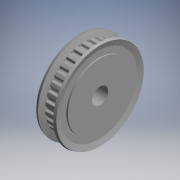
# Autodesk Inventor part: ATP30XL025-A-H10_b
Saved by Autodesk Inventor 2017.3 (Build 213256000, 256)
## iProperties
Part Number: ATP30XL025-A-H10_b
Material: Generic
Catalog Web Link: www.cadenas.de
Description: ATP__XL025, ATP__XL031, ATP__ XL037, ATP__XL050, BTP__XL025, BTP__XL031, BTP__XL037, BTP__XL050, KTP__XL025, KTP__XL031, KTP__ XL037, KTP__XL050, NTP__XL025, NTP__XL031, NTP__ XL037, NTP__XL050, MTP__XL025, MTP__ XL037, MTP__XL050, MTPB__XL025, MTPB__ XL037, MTPB__XL050, MTPP__XL025, MTPP__ XL037, MTPP__XL050, STP__XL025, STP__ XL037, STP__XL050_body-Timing Pulleys XL Type
Vendor: MISUMI
Document SubType Name: Modeling
Designer: partserver
Manufacturer: MISUMI
Mass: 21.798 g
Surface Area: 84.2967 cm^2
Volume: 21.798 cm^3
Density: 1 g/cm^3
Appearance: PSOLRGB-192-192-192
Category: PARTsolutions
Company: MISUMI
Title: ATP30XL025-A-H10
Author: Cadenas PARTsolutions
Comments: Timing Pulleys XL Type
PSOL_IDENT_0: {$CADENAS_DATA\23d-libs\misumi\metric\51_timing_pulleys\mtp_xl\mtp_xl.prj},758 {VTYP=3D},{NB=ATP30XL
PSOL_IDENT_1: 025-A-H10_b},{LINA=ATP30XL025-A-H10},{NN=ATP__XL025, ATP__XL031, ATP__ XL037, ATP__XL050, BTP__XL025
PSOL_IDENT_2: , BTP__XL031, BTP__XL037, BTP__XL050, KTP__XL025, KTP__XL031, KTP__ XL037, KTP__XL050, NTP__XL025, N
PSOL_IDENT_3: TP__XL031, NTP__ XL037, NTP__XL050, MTP__XL025, MTP__ XL037, MTP__XL050, MTPB__XL025, MTPB__ XL037,
PSOL_IDENT_4: MTPB__XL050, MTPP__XL025, MTPP__ XL037, MTPP__XL050, STP__XL025, STP__ XL037, STP__XL050_body},{DATE=
PSOL_IDENT_5: 18.04.2019 05:28:45},{GEOMDATE=08.04.2019 09:29:40},{VERSION=},{LINEID=160},{WBVAR=MATP,ST,TNW,PS,SB
PSOL_IDENT_6: S,DD,Z,J,Q,R,S,T,ALT1,ALT2,M,QSC,QFC,QTC,ALT3,K,KSC,KFC,KTC,ALT4,ZM,ZSC,ZFC,ZTC,ALT5,ALT6,ALT7,FC,AL
PSOL_IDENT_7: T8,SRG,ALT9,BTC,TL,ALT10,TPC,ALT11,BC,ALT12,SLH},{WBNUMERIC=DD,Z,J,Q,R,S,T,QSC,QFC,QTC,K,KSC,KFC,KTC
PSOL_IDENT_8: ,ZSC,ZFC,ZTC,FC,SRG,BTC,TL,BC,SLH}  {NB=ATP30XL025-A-H10_b},{LINA=ATP30XL025-A-H10},{KT=DUMMY},{PN=A
PSOL_IDENT_9: TP30XL025-A-H10},{TYPE=ATP},{MATP=A2017},{MATPALG= 'A2017','Aluminum Alloy 2000 series','S45C','1045
PSOL_IDENT_10: Carbon Steel Equivalent','SUS304','SUS304' },{ST=CA},{STALG= 'CA','Clear Anodize','BA','Black Anodi
PSOL_IDENT_11: ze','HAT','Hard Clear Anodize','ENP','Electroless Nickel Plating' },{NT=30},{TNW=XL025},{TNWALG= 'XL
PSOL_IDENT_12: 025','XL031','XL037','XL050' },{BW=6.4mm (1/4inch)},{PS=A},{PSALG= 'A','B' },{SBS=H},{SBSALG= 'H','R
PSOL_IDENT_13: ound Hole','P','Round Hole + Tap','N','New JIS Keywayed Bore + Tap (Standard)','NK','New JIS Keywaye
PSOL_IDENT_14: d Bore + Tap (width 4.0mm, height 1.8mm)','C','Old JIS Keywayed Bore + Tap','V','Stepped Hole','Y','
PSOL_IDENT_15: Both Ends Stepped Hole','WB','Double Stepped Hole' },{DD=10.00},{DDALG=[10:12/1],12.7,[13:36/1]},{DD
PSOL_IDENT_16: HA=[10:12/1],12.7,[13:36/1]},{DDPA=[10:12/1],12.7,[13:31/1]},{DDNA=[10:30/1]},{DDNK=[10:10/1]},{DDCA=
PSOL_IDENT_17: [10,12,15,16,18,19,20]},{DDVA=[10:12/1],12.7,[13:34/1]},{DDY=[10:34/1]},{DDWB=[10:32/1]},{DDHB=},{DD
PSOL_IDENT_18: PB=},{DDNB=},{DDCB=},{DDVFB=},{Z=0},{ZALG=[0]},{ZMIN=12.000},{ZAMAX=36.000},{ZBMAX=0.000},{DDZ=10.00
PSOL_IDENT_19: 0},{J=0.0},{JALG=[0]},{JMIN=2.000},{JMAX=10.5},{JPN=},{Q=0},{QALG=[0]},{QRMIN=12.000},{QRMAX=36},{WB
PSOL_IDENT_20: QMIN=14.000},{R=0},{RALG=[0]},{WBRMAX=-2.000},{S=0.0},{SALG=[0]},{SMAX=6.5},{T=0.0},{TALG=[0]},{TMAX=
PSOL_IDENT_21: 8},{SBSPN=-H10},{A=7.5},{W=12.5},{L=0},{PD=48.51},{OD=48.00},{D=0},{DALG=35.000},{DE=40},{F=55},{E=4
PSOL_IDENT_22: 0},{TT=1.6},{BBK=0.000},{TTK=0.0},{ALT1=},{ALT1ALG= '','Not applicable' },{ANG=120.000},{ALT1PN=},{A
PSOL_IDENT_23: LT2=},{ALT2ALG= '','w/o Side Tapped Hole','QSC','with QSC (6 Places Side Tapped Hole)','QFC','with Q
PSOL_IDENT_24: FC (4 Places Side Tapped Hole)','QTC','with QTC (3 Places Side Tapped Hole)' },{M=N/A},{MALG= 'N/A'
PSOL_IDENT_25: },{MFTALG= 'N/A' },{MSALG= 'N/A' },{M3D=0.000},{KDML=0.000},{ML=0.000},{MUL=0.000},{PITCH=0.000},{QS
PSOL_IDENT_26: C=0.0},{QSCALG=0},{QFC=0.0},{QFCALG=0},{QTC=0.0},{QTCALG=0},{QPCDMIN=0.000},{QPCDMINALG=0.000},{QPCD
PSOL_IDENT_27: MAX=36.000},{ALT2PN=},{TAP=0.000},{ALT3=},{ALT3ALG= '','w/o Side Through Hole','KSC','with KSC (6 Pl
PSOL_IDENT_28: aces Side Through Hole)','KFC','with KFC (4 Places Side Through Hole)','KTC','with KTC (3 Places Sid
PSOL_IDENT_29: e Through Hole)' },{K=0.0},{KALG=0},{KMIN=4.000},{KFTMAX=11.000},{KSMAX=10.500},{KSC=0.0},{KSCALG=0}
PSOL_IDENT_30: ,{KFC=0.0},{KFCALG=0},{KTC=0.0},{KTCALG=0},{KSCMIN=14.000},{KPCDMIN=14.000},{KPCDMAX=36.000},{ALT3PN=
PSOL_IDENT_31: },{ALT4=},{ALT4ALG= '','w/o Side Counterbored','ZSC','with ZSC (6 Places Side Counterbored)','ZFC','
PSOL_IDENT_32: with ZFC (4 Places Side Counterbored)','ZTC','with ZTC (3 Places Side Counterbored)' },{ALT4MIN=20.5
PSOL_IDENT_33: 00},{ALT4MAX=29.500},{ZM=N/A},{ZMALG= 'N/A' },{ZMFTALG= 'N/A' },{ZMSALG= 'N/A' },{ZMDD1=0.0},{ZMDD2=
PSOL_IDENT_34: 0.0},{ZMHH=0.0},{ZSC=0.0},{ZSCALG=[0]},{ZFC=0.0},{ZFCALG=[0]},{ZTC=0.0},{ZTCALG=[0]},{ZPCDMIN=0.000}
PSOL_IDENT_35: ,{ZPCDMINALG=0.000},{ZPCDMAX=36.000},{ALT4PN=},{ALT5=},{ALT5ALG= '','w/o Flange not Attached','NFC','
PSOL_IDENT_36: with NFC (Flange not Attached)' },{ALT5PN=},{ALT6=},{ALT6ALG= '','w/o Flange Attached on One Side On
PSOL_IDENT_37: ly','RFC','with RFC (Flange Attached on The Boss Side Only)','LFC','with LFC (Flange Attached on The
PSOL_IDENT_38: Opposite Side Only)' },{ALT6PN=},{ALT7=},{ALT7ALG= '','w/o FC (Flange Cut)','FC','with FC (Flange C
PSOL_IDENT_39: ut)' },{FC=0.0},{FCALG=0},{FCMIN=49.0},{FCMAX=53.0},{ALT7PN=},{ALT8=},{ALT8ALG= '','Not applicable'
PSOL_IDENT_40: },{ALT8ALGALG=36.000},{ALT8DD2=0.000},{ALT8MM=0.000},{ALT8NN=0.000},{QC=0.000},{KC=0.000},{ZC=0.000}
PSOL_IDENT_41: ,{SRG=0.0},{SRGALG=[0]},{SRGMAX=0.000},{DD2=0.0},{MM=0.00},{NN=0.00},{ALT8PN=},{ALT9=},{ALT9ALG= '','
PSOL_IDENT_42: w/o BTC (Taper for Bearing Holder)','BTC','with BTC (Taper for Bearing Holder)' },{BTC9=11.000},{TL9=
PSOL_IDENT_43: 1.000},{BTC=0},{BTCALG=[0]},{TL=0.0},{TLALG=0},{TLMIN=1.000},{TLMAX=-13.000},{BTCL=0},{BTCD=0},{ALT9
PSOL_IDENT_44: PN=},{WLBCTL=12.500},{ALT10=},{ALT10ALG= '','Not applicable' },{TPC=N/A},{TPCALG= 'N/A' },{TPCM=4.00
PSOL_IDENT_45: 0},{ALT10PN=},{ALT11=},{ALT11ALG= '','Not applicable' },{BC=0.0},{BCALG=0},{BCMIN=3},{BCMAX=-13},{M1
PSOL_IDENT_46: WBC=6.25},{ALT11PN=},{KTT=19},{ALT12=},{ALT12ALG= '','Not applicable' },{SLH=0},{SLHALG=[0]},{ALT12P
PSOL_IDENT_47: N=},{AC=-},{M1=4.000},{M1L=3.000},{KEYA=0.000},{KEYB=0.000},{KEYM=0.000}
NB: ATP30XL025-A-H10_b
NN: 0
NT: 30
NBSYN: $PN._b
LINA: ATP30XL025-A-H10
CATALOG: Misumi
PN: ATP30XL025-A-H10
MATP: Aluminum Alloy 2000 series
ST: Clear Anodize
TNW: XL025
BW: 6.4mm (1/4inch)
PS: A
SBS: Round Hole
DD: 10
Z: 0
J: 0
Q: 0
R: 0
S: 0
T: 0
A: 7.5
W: 12.5
L: 0
PD: 48.51
OD: 48
D: 0
F: 55
E: 40
TT: 1.6
ALT1: Not applicable
ALT2: w/o Side Tapped Hole
M: N/A
QSC: 0
QFC: 0
QTC: 0
ALT3: w/o Side Through Hole
K: 0
KSC: 0
KFC: 0
KTC: 0
ALT4: w/o Side Counterbored
ZM: N/A
ZMDD1: 0
ZMDD2: 0
ZMHH: 0
ZSC: 0
ZFC: 0
ZTC: 0
ALT5: w/o Flange not Attached
ALT6: w/o Flange Attached on One Side Only
ALT7: w/o FC (Flange Cut)
FC: 0
ALT8: Not applicable
SRG: 0
DD2: 0
MM: 0
ALT9: w/o BTC (Taper for Bearing Holder)
BTC: 0
TL: 0
BTCL: 0
BTCD: 0
ALT10: Not applicable
TPC: N/A
ALT11: Not applicable
BC: 0
ALT12: Not applicable
SLH: 0
AC: -
SUPPLIER: MISUMI
ARTICLENO: ATP30XL025-A-H10_b
BOMINFO: ATP30XL025-A-H10
CREATOR: CADENAS GmbH
Autodesk Inventor part; units mm, degrees
ref_plane "YZ Plane" through (0, 0, 0) normal (1, 0, 0) x (0, 1, 0)
ref_plane "XZ Plane" through (0, 0, 0) normal (0, 1, 0) x (-1, 0, 0)
ref_plane "XY Plane" through (0, 0, 0) normal (0, 0, 1) x (1, 0, 0)
sketch "_____2" plane through (0, 0, 0) normal (0, 0, 1) x (1, 0, 0)
  line L0 (12.5, 0) -> (0, 0)
  line L1 (0, 0) -> (0, 20)
  line L2 (0, 20) -> (0.9, 20)
  line L3 (0.9, 20) -> (0.9, 23.789356)
  line L4 (0.9, 23.789356) -> (0.016697, 27.08589)
  line L5 (0.016697, 27.08589) -> (1.562178, 27.5)
  line L6 (1.562178, 27.5) -> (2.5, 24)
  line L7 (2.5, 24) -> (10, 24)
  line L8 (10, 24) -> (10.937822, 27.5)
  line L9 (10.937822, 27.5) -> (12.483303, 27.08589)
  line L10 (12.483303, 27.08589) -> (11.6, 23.789356)
  line L11 (11.6, 23.789356) -> (11.6, 20)
  line L12 (11.6, 20) -> (12.5, 20)
  line L13 (12.5, 20) -> (12.5, 0)
  line L14 (12.5, 0) -> (0, 0)
  constraints: 30 end point
revolve "Revolution1" add sketch "_____2" angle 360 about axis through (12.5, 0, 0) along (1, 0, 0)
sketch "Sketch2" plane through (12.5, 0, 0) normal (1, 0, 0) x (0, 0, -1)
  point P0 (0, 0)
hole "Hole1" at (12.5, 0, 0) direction (-1, 0, 0) diameter 10 depth 12.5
sketch "_____6" plane through (2.5, 0, 0) normal (1, 0, 0) x (0, 0, -1)
  arc A0 (-24.255, 0) -> (-23.72497, -5.042898) centre (0, 0) ccw
  arc A1 (-23.72497, -5.042898) -> (-22.158045, -9.865397) centre (0, 0) ccw
  arc A2 (-22.158045, -9.865397) -> (-19.622707, -14.256731) centre (0, 0) ccw
  arc A3 (-19.622707, -14.256731) -> (-16.229763, -18.024978) centre (0, 0) ccw
  arc A4 (-16.229763, -18.024978) -> (-12.1275, -21.005446) centre (0, 0) ccw
  arc A5 (-12.1275, -21.005446) -> (-7.495207, -23.067876) centre (0, 0) ccw
  arc A6 (-7.495207, -23.067876) -> (-2.535338, -24.122129) centre (0, 0) ccw
  arc A7 (-2.535338, -24.122129) -> (2.535338, -24.122129) centre (0, 0) ccw
  arc A8 (2.535338, -24.122129) -> (7.495207, -23.067876) centre (0, 0) ccw
  arc A9 (7.495207, -23.067876) -> (12.1275, -21.005446) centre (0, 0) ccw
  arc A10 (12.1275, -21.005446) -> (16.229763, -18.024978) centre (0, 0) ccw
  arc A11 (16.229763, -18.024978) -> (19.622707, -14.256731) centre (0, 0) ccw
  arc A12 (19.622707, -14.256731) -> (22.158045, -9.865397) centre (0, 0) ccw
  arc A13 (22.158045, -9.865397) -> (23.72497, -5.042898) centre (0, 0) ccw
  arc A14 (23.72497, -5.042898) -> (24.255, 0) centre (0, 0) ccw
  arc A15 (24.255, 0) -> (23.72497, 5.042898) centre (0, 0) ccw
  arc A16 (23.72497, 5.042898) -> (22.158045, 9.865397) centre (0, 0) ccw
  arc A17 (22.158045, 9.865397) -> (19.622707, 14.256731) centre (0, 0) ccw
  arc A18 (19.622707, 14.256731) -> (16.229763, 18.024978) centre (0, 0) ccw
  arc A19 (16.229763, 18.024978) -> (12.1275, 21.005446) centre (0, 0) ccw
  arc A20 (12.1275, 21.005446) -> (7.495207, 23.067876) centre (0, 0) ccw
  arc A21 (7.495207, 23.067876) -> (2.535338, 24.122129) centre (0, 0) ccw
  arc A22 (2.535338, 24.122129) -> (-2.535338, 24.122129) centre (0, 0) ccw
  arc A23 (-2.535338, 24.122129) -> (-7.495207, 23.067876) centre (0, 0) ccw
  arc A24 (-7.495207, 23.067876) -> (-12.1275, 21.005446) centre (0, 0) ccw
  arc A25 (-12.1275, 21.005446) -> (-16.229763, 18.024978) centre (0, 0) ccw
  arc A26 (-16.229763, 18.024978) -> (-19.622707, 14.256731) centre (0, 0) ccw
  arc A27 (-19.622707, 14.256731) -> (-22.158045, 9.865397) centre (0, 0) ccw
  arc A28 (-22.158045, 9.865397) -> (-23.72497, 5.042898) centre (0, 0) ccw
  arc A29 (-23.72497, 5.042898) -> (-24.255, 0) centre (0, 0) ccw
  arc A30 (-24, 0) -> (-23.986149, -0.815261) centre (0, 0) ccw
  arc A31 (-23.986149, -0.815261) -> (-23.575098, -1.371306) centre (-23.376501, -0.79454) ccw
  line L0 (-23.575098, -1.371306) -> (-22.909042, -1.600647)
  arc A32 (-22.500329, -2.120187) -> (-22.909042, -1.600647) centre (-23.107639, -2.177414) ccw
  arc A33 (-22.500329, -2.120187) -> (-22.449455, -2.604225) centre (0, 0) ccw
  arc A34 (-22.741218, -3.197388) -> (-22.449455, -2.604225) centre (-23.055391, -2.674516) ccw
  line L1 (-22.741218, -3.197388) -> (-23.345036, -3.560199)
  arc A35 (-23.345036, -3.560199) -> (-23.631496, -4.189555) centre (-23.030863, -4.083071) ccw
  arc A36 (-23.631496, -4.189555) -> (-23.475542, -4.989881) centre (0, 0) ccw
  arc A37 (-23.475542, -4.989881) -> (-23.292492, -5.784446) centre (0, 0) ccw
  arc A38 (-23.292492, -5.784446) -> (-22.774815, -6.242878) centre (-22.700474, -5.637425) ccw
  line L2 (-22.774815, -6.242878) -> (-22.075631, -6.328727)
  arc A39 (-21.567831, -6.751938) -> (-22.075631, -6.328727) centre (-22.149972, -6.93418) ccw
  arc A40 (-21.567831, -6.751938) -> (-21.417431, -7.21482) centre (0, 0) ccw
  arc A41 (-21.579493, -7.855683) -> (-21.417431, -7.21482) centre (-21.995512, -7.409557) ccw
  line L3 (-21.579493, -7.855683) -> (-22.094684, -8.336106)
  arc A42 (-22.094684, -8.336106) -> (-22.244034, -9.011268) centre (-21.678665, -8.782231) ccw
  arc A43 (-22.244034, -9.011268) -> (-21.925091, -9.761679) centre (0, 0) ccw
  arc A44 (-21.925091, -9.761679) -> (-21.580841, -10.500824) centre (0, 0) ccw
  arc A45 (-21.580841, -10.500824) -> (-20.979163, -10.841607) centre (-21.032328, -10.233928) ccw
  line L4 (-20.979163, -10.841607) -> (-20.27741, -10.780211)
  arc A46 (-19.692715, -11.088596) -> (-20.27741, -10.780211) centre (-20.224245, -11.38789) ccw
  arc A47 (-19.692715, -11.088596) -> (-19.449364, -11.510094) centre (0, 0) ccw
  arc A48 (-19.474641, -12.170646) -> (-19.449364, -11.510094) centre (-19.974324, -11.820765) ccw
  line L5 (-19.474641, -12.170646) -> (-19.878688, -12.747685)
  arc A49 (-19.878688, -12.747685) -> (-19.884401, -13.439145) centre (-19.379005, -13.097567) ccw
  arc A50 (-19.884401, -13.439145) -> (-19.416408, -14.106846) centre (0, 0) ccw
  arc A51 (-19.416408, -14.106846) -> (-18.926004, -14.758265) centre (0, 0) ccw
  arc A52 (-18.926004, -14.758265) -> (-18.266621, -14.966505) centre (-18.444968, -14.383159) ccw
  line L6 (-18.266621, -14.966505) -> (-17.592968, -14.760548)
  arc A53 (-16.956934, -14.940629) -> (-17.592968, -14.760548) centre (-17.414621, -15.343894) ccw
  arc A54 (-16.956934, -14.940629) -> (-16.631265, -15.302321) centre (0, 0) ccw
  arc A55 (-16.518654, -15.953694) -> (-16.631265, -15.302321) centre (-17.080162, -15.715348) ccw
  line L7 (-16.518654, -15.953694) -> (-16.793898, -16.602129)
  arc A56 (-16.793898, -16.602129) -> (-16.655724, -17.279666) centre (-16.23239, -16.840475) ccw
  arc A57 (-16.655724, -17.279666) -> (-16.059135, -17.835476) centre (0, 0) ccw
  arc A58 (-16.059135, -17.835476) -> (-15.444009, -18.370699) centre (0, 0) ccw
  arc A59 (-15.444009, -18.370699) -> (-14.75574, -18.437295) centre (-15.051474, -17.903777) ccw
  line L8 (-14.75574, -18.437295) -> (-14.139629, -18.095778)
  arc A60 (-13.480053, -18.139685) -> (-14.139629, -18.095778) centre (-13.843895, -18.629296) ccw
  arc A61 (-13.480053, -18.139685) -> (-13.086301, -18.425763) centre (0, 0) ccw
  arc A62 (-12.840722, -19.039489) -> (-13.086301, -18.425763) centre (-13.439515, -18.923095) ccw
  line L9 (-12.840722, -19.039489) -> (-12.975135, -19.730981)
  arc A63 (-12.975135, -19.730981) -> (-12.699111, -20.364984) centre (-12.376342, -19.847374) ccw
  arc A64 (-12.699111, -20.364984) -> (-12, -20.78461) centre (0, 0) ccw
  arc A65 (-12, -20.78461) -> (-11.287038, -21.180245) centre (0, 0) ccw
  arc A66 (-11.287038, -21.180245) -> (-10.599963, -21.102287) centre (-11.000159, -20.641914) ccw
  line L10 (-10.599963, -21.102287) -> (-10.06832, -20.640136)
  arc A67 (-9.414028, -20.54595) -> (-10.06832, -20.640136) centre (-9.668124, -21.100509) ccw
  arc A68 (-9.414028, -20.54595) -> (-8.969402, -20.743911) centre (0, 0) ccw
  arc A69 (-8.601589, -21.293167) -> (-8.969402, -20.743911) centre (-9.211497, -21.303813) ccw
  line L11 (-8.601589, -21.293167) -> (-8.589295, -21.997493)
  arc A70 (-8.589295, -21.997493) -> (-8.187487, -22.560254) centre (-7.979388, -21.986847) ccw
  arc A71 (-8.187487, -22.560254) -> (-7.416408, -22.825356) centre (0, 0) ccw
  arc A72 (-7.416408, -22.825356) -> (-6.636768, -23.064113) centre (0, 0) ccw
  arc A73 (-6.636768, -23.064113) -> (-5.980916, -22.845007) centre (-6.468084, -22.4779) ccw
  line L12 (-5.980916, -22.845007) -> (-5.556977, -22.282421)
  arc A74 (-4.936566, -22.054258) -> (-5.556977, -22.282421) centre (-5.06981, -22.649528) ccw
  arc A75 (-4.936566, -22.054258) -> (-4.460498, -22.15545) centre (0, 0) ccw
  arc A76 (-3.986526, -22.616231) -> (-4.460498, -22.15545) centre (-4.580892, -22.753451) ccw
  line L13 (-3.986526, -22.616231) -> (-3.828063, -23.30261)
  arc A77 (-3.828063, -23.30261) -> (-3.31803, -23.769532) centre (-3.233697, -23.16539) ccw
  arc A78 (-3.31803, -23.769532) -> (-2.508683, -23.868525) centre (0, 0) ccw
  arc A79 (-2.508683, -23.868525) -> (-1.69644, -23.939968) centre (0, 0) ccw
  arc A80 (-1.69644, -23.939968) -> (-1.100475, -23.589291) centre (-1.653323, -23.331494) ccw
  line L14 (-1.100475, -23.589291) -> (-0.802768, -22.950857)
  arc A81 (-0.243352, -22.59869) -> (-0.802768, -22.950857) centre (-0.24992, -23.208654) ccw
  arc A82 (-0.243352, -22.59869) -> (0.243352, -22.59869) centre (0, 0) ccw
  arc A83 (0.802768, -22.950857) -> (0.243352, -22.59869) centre (0.24992, -23.208654) ccw
  line L15 (0.802768, -22.950857) -> (1.100475, -23.589291)
  arc A84 (1.100475, -23.589291) -> (1.69644, -23.939968) centre (1.653323, -23.331494) ccw
  arc A85 (1.69644, -23.939968) -> (2.508683, -23.868525) centre (0, 0) ccw
  arc A86 (2.508683, -23.868525) -> (3.31803, -23.769532) centre (0, 0) ccw
  arc A87 (3.31803, -23.769532) -> (3.828063, -23.30261) centre (3.233697, -23.16539) ccw
  line L16 (3.828063, -23.30261) -> (3.986526, -22.616231)
  arc A88 (4.460498, -22.15545) -> (3.986526, -22.616231) centre (4.580892, -22.753451) ccw
  arc A89 (4.460498, -22.15545) -> (4.936566, -22.054258) centre (0, 0) ccw
  arc A90 (5.556977, -22.282421) -> (4.936566, -22.054258) centre (5.06981, -22.649528) ccw
  line L17 (5.556977, -22.282421) -> (5.980916, -22.845007)
  arc A91 (5.980916, -22.845007) -> (6.636768, -23.064113) centre (6.468084, -22.4779) ccw
  arc A92 (6.636768, -23.064113) -> (7.416408, -22.825356) centre (0, 0) ccw
  arc A93 (7.416408, -22.825356) -> (8.187487, -22.560254) centre (0, 0) ccw
  arc A94 (8.187487, -22.560254) -> (8.589295, -21.997493) centre (7.979388, -21.986847) ccw
  line L18 (8.589295, -21.997493) -> (8.601589, -21.293167)
  arc A95 (8.969402, -20.743911) -> (8.601589, -21.293167) centre (9.211497, -21.303813) ccw
  arc A96 (8.969402, -20.743911) -> (9.414028, -20.54595) centre (0, 0) ccw
  arc A97 (10.06832, -20.640136) -> (9.414028, -20.54595) centre (9.668124, -21.100509) ccw
  line L19 (10.06832, -20.640136) -> (10.599963, -21.102287)
  arc A98 (10.599963, -21.102287) -> (11.287038, -21.180245) centre (11.000159, -20.641914) ccw
  arc A99 (11.287038, -21.180245) -> (12, -20.78461) centre (0, 0) ccw
  arc A100 (12, -20.78461) -> (12.699112, -20.364984) centre (0, 0) ccw
  arc A101 (12.699112, -20.364984) -> (12.975135, -19.730981) centre (12.376342, -19.847374) ccw
  line L20 (12.975135, -19.730981) -> (12.840722, -19.039489)
  arc A102 (13.086301, -18.425763) -> (12.840722, -19.039489) centre (13.439515, -18.923095) ccw
  arc A103 (13.086301, -18.425763) -> (13.480052, -18.139686) centre (0, 0) ccw
  arc A104 (14.139629, -18.095778) -> (13.480052, -18.139686) centre (13.843895, -18.629296) ccw
  line L21 (14.139629, -18.095778) -> (14.75574, -18.437295)
  arc A105 (14.75574, -18.437295) -> (15.444009, -18.370699) centre (15.051474, -17.903777) ccw
  arc A106 (15.444009, -18.370699) -> (16.059135, -17.835476) centre (0, 0) ccw
  arc A107 (16.059135, -17.835476) -> (16.655724, -17.279666) centre (0, 0) ccw
  arc A108 (16.655724, -17.279666) -> (16.793898, -16.602129) centre (16.23239, -16.840475) ccw
  line L22 (16.793898, -16.602129) -> (16.518654, -15.953694)
  arc A109 (16.631265, -15.302321) -> (16.518654, -15.953694) centre (17.080162, -15.715348) ccw
  arc A110 (16.631265, -15.302321) -> (16.956933, -14.940629) centre (0, 0) ccw
  arc A111 (17.592968, -14.760548) -> (16.956933, -14.940629) centre (17.414621, -15.343894) ccw
  line L23 (17.592968, -14.760548) -> (18.266621, -14.966505)
  arc A112 (18.266621, -14.966505) -> (18.926004, -14.758265) centre (18.444968, -14.383159) ccw
  arc A113 (18.926004, -14.758265) -> (19.416408, -14.106846) centre (0, 0) ccw
  arc A114 (19.416408, -14.106846) -> (19.884401, -13.439144) centre (0, 0) ccw
  arc A115 (19.884401, -13.439144) -> (19.878688, -12.747685) centre (19.379005, -13.097567) ccw
  line L24 (19.878688, -12.747685) -> (19.474641, -12.170646)
  arc A116 (19.449363, -11.510094) -> (19.474641, -12.170646) centre (19.974324, -11.820765) ccw
  arc A117 (19.449363, -11.510094) -> (19.692715, -11.088596) centre (0, 0) ccw
  arc A118 (20.27741, -10.780211) -> (19.692715, -11.088596) centre (20.224245, -11.38789) ccw
  line L25 (20.27741, -10.780211) -> (20.979163, -10.841607)
  arc A119 (20.979163, -10.841607) -> (21.580841, -10.500824) centre (21.032328, -10.233928) ccw
  arc A120 (21.580841, -10.500824) -> (21.925091, -9.761679) centre (0, 0) ccw
  arc A121 (21.925091, -9.761679) -> (22.244034, -9.011268) centre (0, 0) ccw
  arc A122 (22.244034, -9.011268) -> (22.094684, -8.336106) centre (21.678665, -8.782231) ccw
  line L26 (22.094684, -8.336106) -> (21.579493, -7.855683)
  arc A123 (21.417431, -7.214821) -> (21.579493, -7.855683) centre (21.995512, -7.409557) ccw
  arc A124 (21.417431, -7.214821) -> (21.567831, -6.751938) centre (0, 0) ccw
  arc A125 (22.075631, -6.328727) -> (21.567831, -6.751938) centre (22.149972, -6.93418) ccw
  line L27 (22.075631, -6.328727) -> (22.774815, -6.242878)
  arc A126 (22.774815, -6.242878) -> (23.292492, -5.784446) centre (22.700474, -5.637425) ccw
  arc A127 (23.292492, -5.784446) -> (23.475542, -4.989881) centre (0, 0) ccw
  arc A128 (23.475542, -4.989881) -> (23.631497, -4.189555) centre (0, 0) ccw
  arc A129 (23.631497, -4.189555) -> (23.345036, -3.560199) centre (23.030863, -4.083071) ccw
  line L28 (23.345036, -3.560199) -> (22.741218, -3.197388)
  arc A130 (22.449455, -2.604225) -> (22.741218, -3.197388) centre (23.055391, -2.674516) ccw
  arc A131 (22.449455, -2.604225) -> (22.500329, -2.120187) centre (0, 0) ccw
  arc A132 (22.909042, -1.600647) -> (22.500329, -2.120187) centre (23.107639, -2.177414) ccw
  line L29 (22.909042, -1.600647) -> (23.575098, -1.371306)
  arc A133 (23.575098, -1.371306) -> (23.986149, -0.815261) centre (23.376501, -0.79454) ccw
  arc A134 (23.986149, -0.815261) -> (24, 0) centre (0, 0) ccw
  arc A135 (24, 0) -> (23.986149, 0.815261) centre (0, 0) ccw
  arc A136 (23.986149, 0.815261) -> (23.575098, 1.371306) centre (23.376501, 0.79454) ccw
  line L30 (23.575098, 1.371306) -> (22.909042, 1.600647)
  arc A137 (22.500329, 2.120187) -> (22.909042, 1.600647) centre (23.107639, 2.177414) ccw
  arc A138 (22.500329, 2.120187) -> (22.449455, 2.604225) centre (0, 0) ccw
  arc A139 (22.741218, 3.197388) -> (22.449455, 2.604225) centre (23.055391, 2.674516) ccw
  line L31 (22.741218, 3.197388) -> (23.345036, 3.560199)
  arc A140 (23.345036, 3.560199) -> (23.631497, 4.189555) centre (23.030863, 4.083071) ccw
  arc A141 (23.631497, 4.189555) -> (23.475542, 4.989881) centre (0, 0) ccw
  arc A142 (23.475542, 4.989881) -> (23.292492, 5.784447) centre (0, 0) ccw
  arc A143 (23.292492, 5.784447) -> (22.774815, 6.242878) centre (22.700474, 5.637425) ccw
  line L32 (22.774815, 6.242878) -> (22.075631, 6.328727)
  arc A144 (21.567831, 6.751938) -> (22.075631, 6.328727) centre (22.149972, 6.93418) ccw
  arc A145 (21.567831, 6.751938) -> (21.417431, 7.21482) centre (0, 0) ccw
  arc A146 (21.579493, 7.855683) -> (21.417431, 7.21482) centre (21.995512, 7.409557) ccw
  line L33 (21.579493, 7.855683) -> (22.094684, 8.336106)
  arc A147 (22.094684, 8.336106) -> (22.244034, 9.011268) centre (21.678665, 8.782231) ccw
  arc A148 (22.244034, 9.011268) -> (21.925091, 9.761679) centre (0, 0) ccw
  arc A149 (21.925091, 9.761679) -> (21.580841, 10.500824) centre (0, 0) ccw
  arc A150 (21.580841, 10.500824) -> (20.979163, 10.841607) centre (21.032328, 10.233928) ccw
  line L34 (20.979163, 10.841607) -> (20.27741, 10.780211)
  arc A151 (19.692715, 11.088596) -> (20.27741, 10.780211) centre (20.224245, 11.38789) ccw
  arc A152 (19.692715, 11.088596) -> (19.449364, 11.510094) centre (0, 0) ccw
  arc A153 (19.474641, 12.170646) -> (19.449364, 11.510094) centre (19.974324, 11.820765) ccw
  line L35 (19.474641, 12.170646) -> (19.878688, 12.747685)
  arc A154 (19.878688, 12.747685) -> (19.884401, 13.439145) centre (19.379005, 13.097567) ccw
  arc A155 (19.884401, 13.439145) -> (19.416408, 14.106846) centre (0, 0) ccw
  arc A156 (19.416408, 14.106846) -> (18.926004, 14.758265) centre (0, 0) ccw
  arc A157 (18.926004, 14.758265) -> (18.266621, 14.966505) centre (18.444968, 14.383159) ccw
  line L36 (18.266621, 14.966505) -> (17.592968, 14.760548)
  arc A158 (16.956934, 14.940629) -> (17.592968, 14.760548) centre (17.414621, 15.343894) ccw
  arc A159 (16.956934, 14.940629) -> (16.631265, 15.302321) centre (0, 0) ccw
  arc A160 (16.518654, 15.953694) -> (16.631265, 15.302321) centre (17.080162, 15.715348) ccw
  line L37 (16.518654, 15.953694) -> (16.793898, 16.602129)
  arc A161 (16.793898, 16.602129) -> (16.655724, 17.279666) centre (16.23239, 16.840475) ccw
  arc A162 (16.655724, 17.279666) -> (16.059135, 17.835476) centre (0, 0) ccw
  arc A163 (16.059135, 17.835476) -> (15.444009, 18.370699) centre (0, 0) ccw
  arc A164 (15.444009, 18.370699) -> (14.75574, 18.437295) centre (15.051474, 17.903777) ccw
  line L38 (14.75574, 18.437295) -> (14.139629, 18.095778)
  arc A165 (13.480053, 18.139685) -> (14.139629, 18.095778) centre (13.843895, 18.629296) ccw
  arc A166 (13.480053, 18.139685) -> (13.086301, 18.425763) centre (0, 0) ccw
  arc A167 (12.840722, 19.039489) -> (13.086301, 18.425763) centre (13.439515, 18.923095) ccw
  line L39 (12.840722, 19.039489) -> (12.975135, 19.730981)
  arc A168 (12.975135, 19.730981) -> (12.699111, 20.364984) centre (12.376342, 19.847374) ccw
  arc A169 (12.699111, 20.364984) -> (12, 20.78461) centre (0, 0) ccw
  arc A170 (12, 20.78461) -> (11.287038, 21.180245) centre (0, 0) ccw
  arc A171 (11.287038, 21.180245) -> (10.599963, 21.102287) centre (11.000159, 20.641914) ccw
  line L40 (10.599963, 21.102287) -> (10.06832, 20.640136)
  arc A172 (9.414028, 20.54595) -> (10.06832, 20.640136) centre (9.668124, 21.100509) ccw
  arc A173 (9.414028, 20.54595) -> (8.969402, 20.74391) centre (0, 0) ccw
  arc A174 (8.601589, 21.293167) -> (8.969402, 20.74391) centre (9.211497, 21.303813) ccw
  line L41 (8.601589, 21.293167) -> (8.589295, 21.997493)
  arc A175 (8.589295, 21.997493) -> (8.187487, 22.560254) centre (7.979388, 21.986847) ccw
  arc A176 (8.187487, 22.560254) -> (7.416408, 22.825356) centre (0, 0) ccw
  arc A177 (7.416408, 22.825356) -> (6.636768, 23.064113) centre (0, 0) ccw
  arc A178 (6.636768, 23.064113) -> (5.980916, 22.845007) centre (6.468084, 22.4779) ccw
  line L42 (5.980916, 22.845007) -> (5.556977, 22.282421)
  arc A179 (4.936566, 22.054258) -> (5.556977, 22.282421) centre (5.06981, 22.649528) ccw
  arc A180 (4.936566, 22.054258) -> (4.460498, 22.15545) centre (0, 0) ccw
  arc A181 (3.986526, 22.616231) -> (4.460498, 22.15545) centre (4.580892, 22.753451) ccw
  line L43 (3.986526, 22.616231) -> (3.828063, 23.30261)
  arc A182 (3.828063, 23.30261) -> (3.31803, 23.769532) centre (3.233697, 23.16539) ccw
  arc A183 (3.31803, 23.769532) -> (2.508683, 23.868525) centre (0, 0) ccw
  arc A184 (2.508683, 23.868525) -> (1.69644, 23.939968) centre (0, 0) ccw
  arc A185 (1.69644, 23.939968) -> (1.100475, 23.589291) centre (1.653323, 23.331494) ccw
  line L44 (1.100475, 23.589291) -> (0.802768, 22.950857)
  arc A186 (0.243352, 22.59869) -> (0.802768, 22.950857) centre (0.24992, 23.208654) ccw
  arc A187 (0.243352, 22.59869) -> (-0.243352, 22.59869) centre (0, 0) ccw
  arc A188 (-0.802768, 22.950857) -> (-0.243352, 22.59869) centre (-0.24992, 23.208654) ccw
  line L45 (-0.802768, 22.950857) -> (-1.100475, 23.589291)
  arc A189 (-1.100475, 23.589291) -> (-1.69644, 23.939968) centre (-1.653323, 23.331494) ccw
  arc A190 (-1.69644, 23.939968) -> (-2.508683, 23.868525) centre (0, 0) ccw
  arc A191 (-2.508683, 23.868525) -> (-3.31803, 23.769533) centre (0, 0) ccw
  arc A192 (-3.31803, 23.769533) -> (-3.828063, 23.30261) centre (-3.233697, 23.16539) ccw
  line L46 (-3.828063, 23.30261) -> (-3.986526, 22.616231)
  arc A193 (-4.460497, 22.15545) -> (-3.986526, 22.616231) centre (-4.580892, 22.753451) ccw
  arc A194 (-4.460497, 22.15545) -> (-4.936566, 22.054259) centre (0, 0) ccw
  arc A195 (-5.556977, 22.282421) -> (-4.936566, 22.054259) centre (-5.06981, 22.649528) ccw
  line L47 (-5.556977, 22.282421) -> (-5.980916, 22.845007)
  arc A196 (-5.980916, 22.845007) -> (-6.636768, 23.064113) centre (-6.468084, 22.4779) ccw
  arc A197 (-6.636768, 23.064113) -> (-7.416408, 22.825356) centre (0, 0) ccw
  arc A198 (-7.416408, 22.825356) -> (-8.187487, 22.560254) centre (0, 0) ccw
  arc A199 (-8.187487, 22.560254) -> (-8.589295, 21.997493) centre (-7.979388, 21.986847) ccw
  line L48 (-8.589295, 21.997493) -> (-8.601589, 21.293167)
  arc A200 (-8.969402, 20.743911) -> (-8.601589, 21.293167) centre (-9.211497, 21.303813) ccw
  arc A201 (-8.969402, 20.743911) -> (-9.414028, 20.54595) centre (0, 0) ccw
  arc A202 (-10.06832, 20.640136) -> (-9.414028, 20.54595) centre (-9.668124, 21.100509) ccw
  line L49 (-10.06832, 20.640136) -> (-10.599963, 21.102287)
  arc A203 (-10.599963, 21.102287) -> (-11.287038, 21.180245) centre (-11.000159, 20.641914) ccw
  arc A204 (-11.287038, 21.180245) -> (-12, 20.78461) centre (0, 0) ccw
  arc A205 (-12, 20.78461) -> (-12.699112, 20.364984) centre (0, 0) ccw
  arc A206 (-12.699112, 20.364984) -> (-12.975135, 19.730981) centre (-12.376342, 19.847374) ccw
  line L50 (-12.975135, 19.730981) -> (-12.840722, 19.039489)
  arc A207 (-13.086301, 18.425763) -> (-12.840722, 19.039489) centre (-13.439515, 18.923095) ccw
  arc A208 (-13.086301, 18.425763) -> (-13.480053, 18.139685) centre (0, 0) ccw
  arc A209 (-14.139629, 18.095778) -> (-13.480053, 18.139685) centre (-13.843895, 18.629296) ccw
  line L51 (-14.139629, 18.095778) -> (-14.75574, 18.437295)
  arc A210 (-14.75574, 18.437295) -> (-15.44401, 18.370699) centre (-15.051474, 17.903777) ccw
  arc A211 (-15.44401, 18.370699) -> (-16.059135, 17.835476) centre (0, 0) ccw
  arc A212 (-16.059135, 17.835476) -> (-16.655724, 17.279666) centre (0, 0) ccw
  arc A213 (-16.655724, 17.279666) -> (-16.793898, 16.602129) centre (-16.23239, 16.840475) ccw
  line L52 (-16.793898, 16.602129) -> (-16.518654, 15.953694)
  arc A214 (-16.631265, 15.302321) -> (-16.518654, 15.953694) centre (-17.080162, 15.715348) ccw
  arc A215 (-16.631265, 15.302321) -> (-16.956933, 14.940629) centre (0, 0) ccw
  arc A216 (-17.592968, 14.760548) -> (-16.956933, 14.940629) centre (-17.414621, 15.343894) ccw
  line L53 (-17.592968, 14.760548) -> (-18.266621, 14.966505)
  arc A217 (-18.266621, 14.966505) -> (-18.926004, 14.758265) centre (-18.444968, 14.383159) ccw
  arc A218 (-18.926004, 14.758265) -> (-19.416408, 14.106846) centre (0, 0) ccw
  arc A219 (-19.416408, 14.106846) -> (-19.884401, 13.439144) centre (0, 0) ccw
  arc A220 (-19.884401, 13.439144) -> (-19.878688, 12.747685) centre (-19.379005, 13.097567) ccw
  line L54 (-19.878688, 12.747685) -> (-19.474641, 12.170646)
  arc A221 (-19.449363, 11.510094) -> (-19.474641, 12.170646) centre (-19.974324, 11.820765) ccw
  arc A222 (-19.449363, 11.510094) -> (-19.692715, 11.088596) centre (0, 0) ccw
  arc A223 (-20.27741, 10.780211) -> (-19.692715, 11.088596) centre (-20.224245, 11.38789) ccw
  line L55 (-20.27741, 10.780211) -> (-20.979163, 10.841607)
  arc A224 (-20.979163, 10.841607) -> (-21.580841, 10.500824) centre (-21.032328, 10.233928) ccw
  arc A225 (-21.580841, 10.500824) -> (-21.925091, 9.761679) centre (0, 0) ccw
  arc A226 (-21.925091, 9.761679) -> (-22.244034, 9.011268) centre (0, 0) ccw
  arc A227 (-22.244034, 9.011268) -> (-22.094684, 8.336106) centre (-21.678665, 8.782231) ccw
  line L56 (-22.094684, 8.336106) -> (-21.579493, 7.855683)
  arc A228 (-21.417431, 7.214821) -> (-21.579493, 7.855683) centre (-21.995512, 7.409557) ccw
  arc A229 (-21.417431, 7.214821) -> (-21.567831, 6.751938) centre (0, 0) ccw
  arc A230 (-22.075631, 6.328727) -> (-21.567831, 6.751938) centre (-22.149972, 6.93418) ccw
  line L57 (-22.075631, 6.328727) -> (-22.774815, 6.242878)
  arc A231 (-22.774815, 6.242878) -> (-23.292492, 5.784446) centre (-22.700474, 5.637425) ccw
  arc A232 (-23.292492, 5.784446) -> (-23.475542, 4.989881) centre (0, 0) ccw
  arc A233 (-23.475542, 4.989881) -> (-23.631496, 4.189555) centre (0, 0) ccw
  arc A234 (-23.631496, 4.189555) -> (-23.345036, 3.560199) centre (-23.030863, 4.083071) ccw
  line L58 (-23.345036, 3.560199) -> (-22.741218, 3.197388)
  arc A235 (-22.449455, 2.604225) -> (-22.741218, 3.197388) centre (-23.055391, 2.674516) ccw
  arc A236 (-22.449455, 2.604225) -> (-22.500329, 2.120188) centre (0, 0) ccw
  arc A237 (-22.909042, 1.600647) -> (-22.500329, 2.120188) centre (-23.107639, 2.177414) ccw
  line L59 (-22.909042, 1.600647) -> (-23.575098, 1.371306)
  arc A238 (-23.575098, 1.371306) -> (-23.986149, 0.815261) centre (-23.376501, 0.79454) ccw
  arc A239 (-23.986149, 0.815261) -> (-24, 0) centre (0, 0) ccw
  constraints: 480 point on circle, 240 centre point, 120 end point
extrude "Extrusion1" cut sketch "_____6" along normal blind 7.5
body "Solid1"
